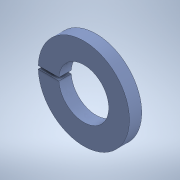
# Autodesk Inventor part: Arandela Grower M8
Saved by Autodesk Inventor 2020 (Build 240168000, 168)
## iProperties
Created: 2020-05-19
Part Number: Arandela Grower M8
Material: Generic
Document SubType Name: Modeling
Designer: Dante
Density: 1 g/cm^3
Appearance: Rubber - Blue
Mass: 0.237656 g
Surface Area: 3.92954 cm^2
Volume: 0.237656 cm^3
Author: Dante
Autodesk Inventor part; units mm, degrees
ref_plane "YZ Plane" through (0, 0, 0) normal (1, 0, 0) x (0, 1, 0)
ref_plane "XZ Plane" through (0, 0, 0) normal (0, 1, 0) x (-1, 0, 0)
ref_plane "XY Plane" through (0, 0, 0) normal (0, 0, 1) x (1, 0, 0)
sketch "Sketch1" plane through (0, 0, 0) normal (0, 0, 1) x (1, 0, 0)
  circle A0 centre (0, 0) radius 4.05
  circle A1 centre (0, 0) radius 7.4
  line L0 (-8.7062, 0.25) -> (-2.7169, 0.25)
  line L1 (-2.7169, -0.25) -> (-8.7062, -0.25)
  line L2 (-8.7062, 0.25) -> (-8.7062, -0.25)
  line L3 (-2.7169, 0.25) -> (-2.7169, -0.25)
  point P0 (-4.0423, -0.25)
  point P1 (-7.3958, -0.25)
  point P2 (-7.3958, 0.25)
  point P3 (-4.0423, 0.25)
  dimension "d0" = 8.1
  dimension "d1" = 14.8
  dimension "d2" = 0.25
  dimension "d3" = 0.5
  constraints: 8 end point, 2 centre point, 2 coincident, 2 horizontal, 2 vertical
  measures "d0" diameter of A0
  measures "d1" diameter of A1
  measures "d2" distance from line of L0 point (0, 0)
  measures "d3" distance between parallel lines of L0 L1
extrude "Extrusion1" add sketch "Sketch1" along normal blind 2 contours A0 L0 A1 L1 picked at (6.1755, 0.9009)
body "Solid1"
